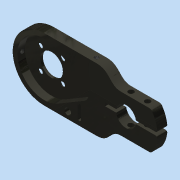
# Autodesk Inventor part: MotorMount
Saved by Autodesk Inventor 2015 (Build 190159000, 159)
## iProperties
Created: 2015-11-05
Part Number: MotorMount
Material: Aluminum 6061
Document SubType Name: Modeling
Designer: Raphael
Density: 2.7 g/cm^3
Appearance: Gunmetal
Mass: 113.033 g
Surface Area: 192.829 cm^2
Volume: 41.8641 cm^3
Author: Raphael
Autodesk Inventor part; units mm, degrees
ref_plane "XZ Plane" through (0, 0, 0) normal (0, 1, 0) x (-1, 0, 0)
ref_plane "XY Plane" through (0, 0, 0) normal (0, 0, 1) x (1, 0, 0)
sketch "Sketch1" plane through (0, 0, 0) normal (0, 0, 1) x (1, 0, 0)
  circle A0 centre (-78.2066, 0) radius 10.75
  arc A1 (-78.2066, 30) -> (-78.2066, -30) centre (-78.2066, 0) ccw
  line L0 (-78.2066, 30) -> (-28.164, 30)
  line L1 (-28.164, -30) -> (-78.2066, -30)
  circle A2 centre (-88.8132, 10.6066) radius 2.1
  circle A3 centre (-67.6, -10.6066) radius 2.1
  circle A4 centre (-88.8132, -10.6066) radius 2.1
  circle A5 centre (-67.6, 10.6066) radius 2.1
  line L2 (-88.8132, 10.6066) -> (-67.6, -10.6066) construction
  line L3 (-67.6, 10.6066) -> (-88.8132, -10.6066) construction
  line L4 (-67.6, 10.6066) -> (-88.8132, 10.6066) construction
  line L5 (-67.6, 10.6066) -> (-67.6, -10.6066) construction
  line L6 (-135.9764, 0) -> (58.4124, 0) projected
  line L7 (9.4315, 1.5) -> (28.2442, 1.5)
  line L8 (28.2442, -1.5) -> (9.4315, -1.5)
  line L9 (-9.4315, 1.5) -> (-29.9625, 1.5)
  line L10 (-9.4315, -1.5) -> (-29.9625, -1.5)
  line L11 (-20, -1.5) -> (-20, 1.5)
  line L12 (9.55, -26.0565) -> (9.55, -21.3339)
  line L13 (12.725, -18.1589) -> (22.25, -18.1589)
  arc A6 (12.725, -18.1589) -> (9.55, -21.3339) centre (12.725, -21.3339) ccw
  arc A7 (7.1295, 29.1405) -> (0, 30) centre (0, 0) ccw
  arc A8 (9.4315, 1.5) -> (-9.4315, 1.5) centre (0, 0) ccw
  arc A9 (-9.4315, -1.5) -> (9.4315, -1.5) centre (0, 0) ccw
  arc A10 (24.8835, -16.7574) -> (29.8223, -3.26) centre (0, 0) ccw
  arc A11 (22.25, -18.1589) -> (24.8835, -16.7574) centre (22.25, -14.9839) ccw
  arc A12 (7.1295, -29.1405) -> (9.55, -26.0565) centre (6.375, -26.0565) ccw
  line L14 (9.55, 26.0565) -> (9.55, 21.3339)
  line L15 (12.725, 18.1589) -> (22.25, 18.1589)
  arc A13 (9.55, 21.3339) -> (12.725, 18.1589) centre (12.725, 21.3339) ccw
  arc A14 (29.8223, 3.26) -> (24.8835, 16.7574) centre (0, 0) ccw
  arc A15 (24.8835, 16.7574) -> (22.25, 18.1589) centre (22.25, 14.9839) ccw
  arc A16 (9.55, 26.0565) -> (7.1295, 29.1405) centre (6.375, 26.0565) ccw
  arc A17 (0, -30) -> (7.1295, -29.1405) centre (0, 0) ccw
  arc A18 (0, 30) -> (0, -30) centre (0, 0) ccw construction
  line L16 (-28.164, -30) -> (-14.7272, -30) construction
  line L17 (-14.7272, -30) -> (-16.1546, -18.1589) construction
  line L18 (-16.1546, -18.1589) -> (-4.7625, -18.1589) construction
  spline S0 degree 3 poles (-28.164, -30) (-14.7272, -30) (-16.1546, -18.1589) (-4.7625, -18.1589) knots 1 1 1 1 2 2 2 2
  arc A19 (28.2442, 1.5) -> (29.8223, 3.26) centre (28.2442, 3.0875) ccw
  arc A20 (29.8223, -3.26) -> (28.2442, -1.5) centre (28.2442, -3.0875) ccw
  line L19 (12.725, -18.1589) -> (-4.7625, -18.1589)
  line L20 (-28.164, 30) -> (-14.7272, 30) construction
  line L21 (-14.7272, 30) -> (-16.1546, 18.1589) construction
  line L22 (-16.1546, 18.1589) -> (-4.7625, 18.1589) construction
  spline S1 degree 3 poles (-28.164, 30) (-14.7272, 30) (-16.1546, 18.1589) (-4.7625, 18.1589) knots 1 1 1 1 2 2 2 2
  line L23 (12.725, 18.1589) -> (-4.7625, 18.1589)
  point P0 (-78.2066, 0)
  point P1 (9.55, -28.4394)
  point P2 (9.55, -18.1589)
  point P3 (23.88, -18.1589)
  point P4 (23.88, -18.1589)
  point P5 (29.9625, -1.5)
  point P6 (9.55, 28.4394)
  point P7 (9.55, 18.1589)
  point P8 (23.88, 18.1589)
  point P9 (23.88, 18.1589)
  point P10 (29.9625, 1.5)
  dimension "d2" = 21.5
  dimension "d3" = 78.2066
  dimension "d4" = 60
  dimension "d5" = 4.2
  dimension "d6" = 4.2
  dimension "d7" = 4.2
  dimension "d8" = 4.2
  dimension "d9" = 30
  dimension "d13" = 3
  dimension "d20" = 3
  dimension "d21" = 1.5
  dimension "d22" = 20
  dimension "d34" = 3.175
  dimension "d35" = 30
  dimension "d38" = 9.55
  dimension "d39" = 9.55
  dimension "d41" = 30
  dimension "d43" = 3.175
  dimension "d44" = 9.525
  dimension "d45" = 3.175
  dimension "d49" = 1.5875
  dimension "d85" = 4.7625
  constraints: 46 point on circle, 36 end point, 21 centre point, 20 tangent, 17 symmetric about line, 15 point on line, 4 coincident, 4 horizontal, 4 perpendicular, 3 parallel, 3 vertical alignment, 2 horizontal alignment, 2 midpoint, 1 equal radius, 1 vertical, 11 other
  measures "d2" diameter of A0
  measures "d3" distance of A0.centre point (0, 0)
  measures "d4" diameter of A1
  measures "d5" diameter of A2
  measures "d6" diameter of A3
  measures "d7" diameter of A4
  measures "d8" diameter of A5
  measures "d9" distance of L3.start L3.end
  measures "d13" distance between parallel lines of L7 L8
  measures "d20" distance between parallel lines of L9 L10
  measures "d21" distance between parallel lines of L6 L9
  measures "d22" distance from line of A8.centre L11
  measures "d34" radius of A6
  measures "d35" radius of A7
  measures "d38" radius of A8
  measures "d39" radius of A9
  measures "d41" radius of A10
  measures "d43" radius of A11
  measures "d44" distance of L13.start L13.end
  measures "d45" radius of A12
  measures "d49" radius of A19
  measures "d85" horizontal distance of L18.end point (0, 0)
extrude "Extrusion4" add sketch "Sketch1" along normal blind 9.525 contours L6 L11 L10 A9 L8 A20 A10 A11 L13 L19 S0 L1 A1 A0 | A0 L6 A1 L0 S1 L23 L15 A15 A14 A19 L7 A8 L9 L11
sketch "Sketch4" plane through (0, 0, 9.525) normal (0, 0, 1) x (1, 0, 0)
  circle A0 centre (-78.2066, 0) radius 10.75 projected
  arc A1 (-65.2016, 21.9344) -> (-65.2016, -21.9344) centre (-78.2066, 0) ccw
  line L0 (-65.2016, 21.9344) -> (-39.7222, 6.8276)
  line L1 (-39.7222, -6.8276) -> (-65.2016, -21.9344)
  line L2 (-135.8143, 0) -> (57.4394, 0) projected
  arc A2 (-39.7222, -6.8276) -> (-39.7222, 6.8276) centre (-43.7703, 0) ccw
  point P0 (0, 0)
  point P1 (-28.2066, 0)
  dimension "d28" = 51
  dimension "d29" = 50
  dimension "d30" = 7.9375
  constraints: 4 end point, 4 point on circle, 4 tangent, 3 point on line, 2 centre point, 1 coincident
  measures "d28" diameter of A1
  measures "d29" distance of point (-28.207, 0) A0.centre
  measures "d30" radius of A2
extrude "Extrusion6" cut sketch "Sketch4" against normal blind 7.1437 contours L2 A2 L1 A1 A0 | A0 L2 A1 L0 A2
sketch "Sketch5" plane through (12.675, 18.1589, 0) normal (0, 1, 0) x (1, 0, 0)
  line L0 (9.575, 0) -> (9.575, -9.525) construction
  line L1 (-3.2435, 0) -> (-3.2435, -9.525) construction
  line L2 (9.575, 0) -> (-17.4375, 0) projected
  line L3 (9.575, -9.525) -> (-17.4375, -9.525) projected
  line L4 (9.575, 0) -> (-3.2435, 0) construction
  line L5 (-3.2435, -9.525) -> (9.575, -9.525) construction
  circle A0 centre (3.1657, -4.7625) radius 2.5527
  line L6 (-22.1065, 0) -> (-22.1065, -9.525) projected
  line L7 (-22.1065, 0) -> (-3.2435, 0) construction
  circle A1 centre (-12.675, -4.7625) radius 2.5527
  point P0 (-3.2435, -4.7625)
  point P1 (3.1657, 0)
  point P2 (-12.675, 0)
  dimension "d86" = 5.1054
  dimension "d87" = 5.1054
  constraints: 6 end point, 3 midpoint, 2 centre point, 2 collinear, 2 horizontal alignment, 2 vertical alignment, 1 horizontal
  measures "d86" diameter of A0
  measures "d87" diameter of A1
extrude "Extrusion7" cut sketch "Sketch5" against normal through all
sketch "Sketch6" plane through (-78.2066, 30, 0) normal (0, 1, 0) x (1, 0, 0)
  line L0 (50.0426, 0) -> (0, 0) projected
  line L1 (0, 0) -> (0, -9.525) projected
  line L2 (50.0426, -9.525) -> (0, -9.525) projected
  line L3 (50.0426, 0) -> (50.0426, -9.525) projected
  circle A0 centre (45.2801, -4.7625) radius 2.0193
  point P0 (78.2066, 0)
  point P1 (50.0426, -4.7625)
  dimension "d50" = 4.0386
  dimension "d51" = 4.7625
  constraints: 1 centre point, 1 horizontal alignment, 1 midpoint
  measures "d50" diameter of A0
  measures "d51" distance of A0.centre point (50.043, -4.763)
extrude "Extrusion8" cut sketch "Sketch6" against normal blind 12.7 contours A0
thread "Thread2" size "10-32 UNF" class "2B" standard "ANSI Unified Screw Threads" full length
mirror "Mirror1" about plane through (0, 0, 0) normal (0, 1, 0) of "Extrusion8"
ref_plane "Work Plane2" through (-108.2066, 0, 0) normal (1, 0, 0) x (0, 1, 0)
sketch "Sketch7" plane through (-108.2066, 0, 0) normal (1, 0, 0) x (0, 1, 0)
  line L0 (30, 0) -> (-30, 0) projected
  line L1 (-30, 0) -> (-30, 9.525) projected
  line L2 (30, 9.525) -> (-30, 9.525) projected
  line L3 (30, 0) -> (30, 9.525) projected
  circle A0 centre (0, 4.7625) radius 2.0193
  point P0 (0, 0)
  point P1 (-30, 4.7625)
  point P2 (0, 9.525)
  dimension "d54" = 4.0386
  constraints: 2 midpoint, 1 centre point, 1 horizontal alignment, 1 vertical alignment
  measures "d54" diameter of A0
extrude "Extrusion9" cut sketch "Sketch7" along normal up to surface contours A0
sketch "Sketch8" plane through (0, 0, 9.525) normal (0, 0, 1) x (1, 0, 0)
  circle A0 centre (-67.6, 10.6066) radius 2.1 projected
  circle A1 centre (-88.8132, -10.6066) radius 2.1 projected
  circle A2 centre (-67.6, -10.6066) radius 2.1 projected
  circle A3 centre (-88.8132, 10.6066) radius 2.1 projected
  circle A4 centre (-78.2066, 0) radius 10.75 projected
  arc A5 (-65.2016, 21.9344) -> (-65.2016, -21.9344) centre (-78.2066, 0) ccw projected
  line L0 (-39.7222, -6.8276) -> (-65.2016, -21.9344) projected
  arc A6 (-39.7222, -6.8276) -> (-39.7222, 6.8276) centre (-43.7703, 0) ccw projected
  line L1 (-65.2016, 21.9344) -> (-39.7222, 6.8276) projected
  line L2 (-39.7222, -6.8276) -> (-65.2016, -21.9344) projected
  arc A7 (-65.2016, 21.9344) -> (-65.2016, -21.9344) centre (-78.2066, 0) ccw projected
  line L3 (-65.2016, 21.9344) -> (-39.7222, 6.8276) projected
  arc A8 (-39.7222, -6.8276) -> (-39.7222, 6.8276) centre (-43.7703, 0) ccw projected
  arc A9 (-78.2066, 30) -> (-78.2066, -30) centre (-78.2066, 0) ccw projected
  line L4 (-78.2066, -30) -> (-28.164, -30) projected
  line L5 (-4.7625, -18.1589) -> (22.25, -18.1589) projected
  arc A10 (22.25, -18.1589) -> (24.8835, -16.7574) centre (22.25, -14.9839) ccw projected
  arc A11 (24.8835, -16.7574) -> (29.8223, -3.26) centre (0, 0) ccw projected
  arc A12 (29.8223, -3.26) -> (28.2442, -1.5) centre (28.2442, -3.0875) ccw projected
  line L6 (28.2442, -1.5) -> (9.4315, -1.5) projected
  arc A13 (-9.4315, -1.5) -> (9.4315, -1.5) centre (0, 0) ccw projected
  line L7 (-9.4315, -1.5) -> (-20, -1.5) projected
  line L8 (-20, -1.5) -> (-20, 1.5) projected
  line L9 (-20, 1.5) -> (-9.4315, 1.5) projected
  arc A14 (9.4315, 1.5) -> (-9.4315, 1.5) centre (0, 0) ccw projected
  line L10 (9.4315, 1.5) -> (28.2442, 1.5) projected
  arc A15 (28.2442, 1.5) -> (29.8223, 3.26) centre (28.2442, 3.0875) ccw projected
  arc A16 (29.8223, 3.26) -> (24.8835, 16.7574) centre (0, 0) ccw projected
  arc A17 (24.8835, 16.7574) -> (22.25, 18.1589) centre (22.25, 14.9839) ccw projected
  line L11 (22.25, 18.1589) -> (-4.7625, 18.1589) projected
  line L12 (-28.164, 30) -> (-78.2066, 30) projected
  circle A18 centre (-55.6441, -23.65) radius 3.175
  line L13 (-135.9764, 0) -> (58.4124, 0) projected
  dimension "d57" = 6.35
  dimension "d58" = 6.35
  dimension "d59" = 6.35
  constraints: 1 centre point, 2 other
  measures "d57" diameter of A18
  measures "d58" distance from line of L4 A18.centre
  measures "d59" distance from line of L0 A18.centre
extrude "Extrusion10" cut sketch "Sketch8" against normal through all contours A18
chamfer "Chamfer1" distance 2.05 angle 45 4 edges at (-69.7, -10.6066, 0) (-69.7, 10.6066, 0) (-90.9132, 10.6066, 0) (-90.9132, -10.6066, 0) measured on face at (-37.888, 14.0355, 0)
sketch "Sketch9" plane through (0, 0, 0) normal (0, 0, -1) x (-1, 0, 0)
  circle A0 centre (78.2066, 0) radius 10.75 projected
  arc A1 (-9.4315, -1.5) -> (9.4315, -1.5) centre (0, 0) ccw projected
  arc A2 (9.4315, 1.5) -> (-9.4315, 1.5) centre (0, 0) ccw projected
  arc A3 (80.5159, -8.2842) -> (80.5159, 8.2842) centre (78.2066, 0) ccw
  arc A4 (7.9482, 28.5129) -> (7.9482, -28.5129) centre (0, 0) ccw
  line L0 (7.9482, 28.5129) -> (80.5159, 8.2842)
  line L1 (80.5159, -8.2842) -> (7.9482, -28.5129)
  circle A5 centre (55.6441, -23.65) radius 3.175 projected
  line L2 (34.9458, -30) -> (30.9072, -30) projected
  circle A6 centre (55.6441, -23.65) radius 3.175 projected
  line L3 (52.4691, -23.65) -> (52.4691, -30) construction
  line L4 (52.4691, -30) -> (34.9458, -30)
  circle A7 centre (44.5012, -22.476) radius 4 construction
  arc A8 (42.9012, -24.476) -> (46.1012, -24.476) centre (44.5012, -24.476) ccw
  arc A9 (46.1012, -13.476) -> (42.9012, -13.476) centre (44.5012, -13.476) ccw
  line L5 (46.1012, -24.476) -> (46.1012, -13.476)
  line L6 (42.9012, -13.476) -> (42.9012, -24.476)
  point P0 (43.7074, -30)
  dimension "d65" = 17.2
  dimension "d66" = 59.2
  dimension "d67" = 8
  dimension "d68" = 3.2
  dimension "d69" = 3.2
  dimension "d70" = 2
  dimension "d71" = 11
  dimension "d84" = 0.7937
  constraints: 12 end point, 8 point on circle, 8 tangent, 5 centre point, 3 vertical, 2 coincident, 2 horizontal alignment, 2 vertical alignment, 1 collinear, 1 midpoint, 2 other
  measures "d65" diameter of A3
  measures "d66" diameter of A4
  measures "d67" diameter of A7
  measures "d68" diameter of A8
  measures "d69" diameter of A9
  measures "d70" distance of A7.centre A8.centre
  measures "d71" distance of A9.centre A8.centre
  measures "d84" horizontal distance of point (43.707, -30) A8.centre
extrude "Extrusion11" cut sketch "Sketch9" against normal through all contours L5 A8 L6 L1 | L1 L6 A9 L5
sketch "Sketch10" plane through (-78.2066, -30, 0) normal (0, -1, 0) x (1, 0, 0)
  line L0 (35.3054, 0) -> (35.3054, 9.525) projected
  line L1 (32.1054, 0) -> (32.1054, 9.525) projected
  circle A0 centre (33.7054, 4.7625) radius 1.25
  line L2 (35.3054, 9.525) -> (32.1054, 9.525) construction
  point P0 (78.2066, 0)
  point P1 (32.1054, 4.7625)
  point P2 (33.7054, 9.525)
  dimension "d74" = 2.5
  constraints: 2 end point, 2 midpoint, 1 centre point, 1 horizontal alignment, 1 perpendicular, 1 vertical alignment
  measures "d74" diameter of A0
extrude "Extrusion12" cut sketch "Sketch10" against normal up to surface
thread "Thread1" size "M3x0.5" class "6H" standard "ANSI Metric M Profile" full length
thread "Thread3" size "10-32 UNF" class "2B" standard "ANSI Unified Screw Threads" full length
equation "\"d3\" = center_distance"
equation "\"d4\" = mount_diameter"
equation "\"d9\" = hole_pattern_diameter"
equation "\"d13\" = clamp_slit"
equation "\"d20\" = clamp_slit"
equation "\"d21\" = 0.5 * clamp_slit"
equation "\"d35\" = 0.5 * mount_diameter"
equation "\"d41\" = 0.5 * mount_diameter"
equation "\"d23\" = thickness"
equation "\"d31\" = thickness - motor_mount_thickness"
equation "\"mount_diameter\" = 60"
equation "\"center_distance\" = 78.2066"
equation "\"hole_pattern_diameter\" = 30"
equation "\"thickness\" = 9.525"
equation "\"clamp_slit\" = 3"
equation "\"motor_mount_thickness\" = 2.38125"
body "Solid2"
